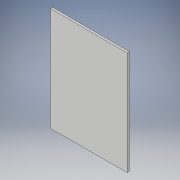
# Autodesk Inventor part: Electronics Plate
Saved by Autodesk Inventor 2017 (Build 210142000, 142)
## iProperties
Created: 2018-04-28
Part Number: Electronics Plate
Material: Generic
Document SubType Name: Modeling
Designer: User
Density: 1 g/cm^3
Appearance: Default
Author: User
Autodesk Inventor part; units mm, degrees
ref_plane "YZ Plane" through (0, 0, 0) normal (1, 0, 0) x (0, 1, 0)
ref_plane "XZ Plane" through (0, 0, 0) normal (0, 1, 0) x (-1, 0, 0)
ref_plane "XY Plane" through (0, 0, 0) normal (0, 0, 1) x (1, 0, 0)
sketch "Sketch1" plane through (0, 0, 0) normal (0, 0, 1) x (1, 0, 0)
  line L0 (-107, -145.0975) -> (107, -145.0975)
  line L1 (107, -145.0975) -> (107, 145.0975)
  line L2 (107, 145.0975) -> (-107, 145.0975)
  line L3 (-107, 145.0975) -> (-107, -145.0975)
  line L4 (-107, -145.0975) -> (107, 145.0975) construction
  line L5 (107, -145.0975) -> (-107, 145.0975) construction
  point P0 (0, 0)
  dimension "d0" = 214
  dimension "d1" = 290.195
  constraints: 12 end point, 2 midpoint, 2 parallel, 1 horizontal, 1 perpendicular
  measures "d0" distance of L2.end L1.end
  measures "d1" distance of L1.end L0.end
extrude "Extrusion1" add sketch "Sketch1" along normal blind 6.35
body "Solid1"
